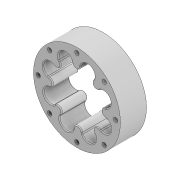
# Autodesk Inventor part: Cycloidal gear inner gear
Saved by Autodesk Inventor 2020.3 (Build 243373010, 373A)
## iProperties
Created: 2021-05-01
Part Number: Cycloidal gear inner gear
Material: Generic
Document SubType Name: Modeling
Designer: marti
Density: 1 g/cm^3
Appearance: Default
Author: marti
Autodesk Inventor part; units mm, degrees
ref_plane "YZ Plane" through (0, 0, 0) normal (1, 0, 0) x (0, 1, 0)
ref_plane "XZ Plane" through (0, 0, 0) normal (0, 1, 0) x (-1, 0, 0)
ref_plane "XY Plane" through (0, 0, 0) normal (0, 0, 1) x (1, 0, 0)
sketch "Sketch2" plane through (0, 0, 0) normal (0, 0, 1) x (1, 0, 0)
  circle A0 centre (0, 0) radius 50
  arc A1 (-5.6574, 32.6914) -> (3.9387, 32.9426) centre (-0.8549, 32.6488) ccw
  arc A2 (-5.6574, 32.6914) -> (-20.5089, 26.079) centre (-13.5131, 30.351) ccw
  arc A3 (-27.1166, 19.1159) -> (-20.5089, 26.079) centre (-23.6907, 22.4816) ccw
  arc A4 (-27.1166, 19.1159) -> (-32.9426, 3.9387) centre (-31.0166, 11.9062) ccw
  arc A5 (-32.6914, -5.6574) -> (-32.9426, 3.9387) centre (-32.6488, -0.8549) ccw
  arc A6 (-32.6914, -5.6574) -> (-26.079, -20.5089) centre (-30.351, -13.5131) ccw
  arc A7 (-19.1159, -27.1166) -> (-26.079, -20.5089) centre (-22.4816, -23.6907) ccw
  arc A8 (-19.1159, -27.1166) -> (-3.9387, -32.9426) centre (-11.9062, -31.0166) ccw
  arc A9 (5.6574, -32.6914) -> (-3.9387, -32.9426) centre (0.8549, -32.6488) ccw
  arc A10 (5.6574, -32.6914) -> (20.5089, -26.079) centre (13.5131, -30.351) ccw
  arc A11 (27.1166, -19.1159) -> (20.5089, -26.079) centre (23.6907, -22.4816) ccw
  arc A12 (27.1166, -19.1159) -> (32.9426, -3.9387) centre (31.0166, -11.9062) ccw
  arc A13 (32.6914, 5.6574) -> (32.9426, -3.9387) centre (32.6488, 0.8549) ccw
  arc A14 (32.6914, 5.6574) -> (26.079, 20.5089) centre (30.351, 13.5131) ccw
  arc A15 (19.1159, 27.1166) -> (26.079, 20.5089) centre (22.4816, 23.6907) ccw
  arc A16 (19.1159, 27.1166) -> (3.9387, 32.9426) centre (11.9062, 31.0166) ccw
  dimension "d6" = 100
  constraints: 32 point on circle, 17 centre point
  measures "d6" diameter of A0
extrude "Extrusion1" add sketch "Sketch2" along normal mid plane 30
sketch "Sketch4" plane through (0, 0, -15) normal (0, 0, -1) x (-1, 0, 0)
  circle A0 centre (0, 0) radius 50 projected
  circle A1 centre (0, 0) radius 42.5
  circle A2 centre (0, 0) radius 42.5
  circle A3 centre (0, 0) radius 42.5
  circle A4 centre (0, 0) radius 42.5
  circle A5 centre (0, 0) radius 42.5
  circle A6 centre (0, 0) radius 42.5
  circle A7 centre (0, 0) radius 42.5
  circle A8 centre (0, 0) radius 42.5
  point P0 (-42.5, 0)
  point P1 (-30.052, 30.052)
  point P2 (0, 42.5)
  point P3 (30.052, 30.052)
  point P4 (42.5, 0)
  point P5 (30.052, -30.052)
  point P6 (0, -42.5)
  point P7 (-30.052, -30.052)
  dimension "d6" = 100
  dimension "d10" = 85
  dimension "d9" = 100
  dimension "d13" = 360
  constraints: 2 horizontal alignment, 2 vertical alignment, 1 coincident, 45 other
  measures "d9" diameter of A0
hole "Hole1" at (42.5, 0, -15) at (30.052, 30.052, -15) at (0, 42.5, -15) at (-30.052, 30.052, -15) at (-42.5, 0, -15) at (-30.052, -30.052, -15) at (0, -42.5, -15) at (30.052, -30.052, -15) direction (0, 0, 1) diameter 4.4587 depth 10 tip angle 118 thread size "M5x0.5" class "6H" standard "ISO Metric profile"
sketch "Sketch5" plane through (0, 0, 15) normal (0, 0, 1) x (1, 0, 0)
  circle A0 centre (0, 0) radius 50 projected
  point P0 (0, 44.5)
  dimension "d6" = 100
  dimension "d33" = 44.5
  constraints: 1 vertical alignment
  measures "d33" distance of point (0, 0) point (0, 44.5)
hole "Hole2" at (0, 44.5, 15) direction (0, 0, -1) diameter 5 depth 8 tip angle 118
pattern_circular "Circular Pattern1" count 8 over 360 about axis through (0, 0, -10) along (0, 0, 1) of "Hole2"
fillet "Fillet2" radius 5 4 edges at (3.9387, 32.9426, 7.5) (3.9387, 32.9426, -7.5) (-5.6574, 32.6914, 7.5) (-5.6574, 32.6914, -7.5)
pattern_circular "Circular Pattern2" count 8 over 360 about axis through (0, 0, -10) along (0, 0, 1) of "Fillet2"
fillet "Fillet3" radius 1 64 edges at (-5.7855, 33.0019, 15) (-0.7292, 27.8478, 15) (4.0504, 33.2595, 15) (14.8437, 38.6692, 15) (19.2449, 27.4268, 15) (19.1758, 20.207, 15) (26.3821, 20.6539, 15) (37.8393, 16.8471, 15) (33.0019, 5.7855, 15) (27.8478, 0.7292, 15) (33.2595, -4.0504, 15) (38.6692, -14.8437, 15) (27.4268, -19.2449, 15) (20.207, -19.1758, 15) (20.6539, -26.3821, 15) (16.8471, -37.8393, 15) (5.7855, -33.0019, 15) (0.7292, -27.8478, 15) (-4.0504, -33.2595, 15) (-14.8437, -38.6692, 15) (-19.2449, -27.4268, 15) (-19.1758, -20.207, 15) (-26.3821, -20.6539, 15) (-37.8393, -16.8471, 15) (-33.0019, -5.7855, 15) (-27.8478, -0.7292, 15) (-33.2595, 4.0504, 15) (-38.6692, 14.8437, 15) (-27.4268, 19.2449, 15) (-20.207, 19.1758, 15) (-20.6539, 26.3821, 15) (-16.8471, 37.8393, 15) (20.6539, -26.3821, -15) (20.207, -19.1758, -15) (27.4268, -19.2449, -15) (38.6692, -14.8437, -15) (33.2595, -4.0504, -15) (27.8478, 0.7292, -15) (33.0019, 5.7855, -15) (37.8393, 16.8471, -15) (26.3821, 20.6539, -15) (19.1758, 20.207, -15) (19.2449, 27.4268, -15) (14.8437, 38.6692, -15) (4.0504, 33.2595, -15) (-0.7292, 27.8478, -15) (-5.7855, 33.0019, -15) (-16.8471, 37.8393, -15) (-20.6539, 26.3821, -15) (-20.207, 19.1758, -15) (-27.4268, 19.2449, -15) (-38.6692, 14.8437, -15) (-33.2595, 4.0504, -15) (-27.8478, -0.7292, -15) (-33.0019, -5.7855, -15) (-37.8393, -16.8471, -15) (-26.3821, -20.6539, -15) (-19.1758, -20.207, -15) (-19.2449, -27.4268, -15) (-14.8437, -38.6692, -15) (-4.0504, -33.2595, -15) (0.7292, -27.8478, -15) (5.7855, -33.0019, -15) (16.8471, -37.8393, -15)
body "Solid1"
